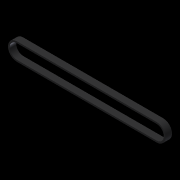
# Autodesk Inventor part: 150T 5mm GT2 Belt
Saved by Autodesk Inventor 2014 SP1 (Build 180222100, 222)
## iProperties
Created: 2013-11-29
Part Number: 150T 5mm GT2 Belt
Material: Rubber, Black
Document SubType Name: Modeling
Designer: Rauhul Varma
Mass: 40.3136 g
Surface Area: 284.75 cm^2
Volume: 43.3479 cm^3
Density: 0.93 g/cm^3
Appearance: Rubber - Black
Author: Rauhul Varma
Autodesk Inventor part; units mm, degrees
ref_plane "YZ Plane" through (0, 0, 0) normal (1, 0, 0) x (0, 1, 0)
ref_plane "XZ Plane" through (0, 0, 0) normal (0, 1, 0) x (-1, 0, 0)
ref_plane "XY Plane" through (0, 0, 0) normal (0, 0, 1) x (1, 0, 0)
sketch "Sketch1" plane through (0, 0, 0) normal (0, 0, 1) x (1, 0, 0)
  arc A0 (0, -16.545) -> (0, 16.545) centre (0, 0) ccw construction
  arc A1 (0, -20.365) -> (0, 20.365) centre (0, 0) ccw construction
  line L0 (0, 0) -> (320.2761, 0) construction
  arc A2 (320.2761, 20.365) -> (320.2761, -20.365) centre (320.2761, 0) ccw construction
  arc A3 (320.2761, 16.545) -> (320.2761, -16.545) centre (320.2761, 0) ccw construction
  line L1 (0, -16.545) -> (320.2761, -16.545)
  line L2 (320.2761, -20.365) -> (0, -20.365)
  line L3 (0, 20.365) -> (320.2761, 20.365)
  line L4 (320.2761, 16.545) -> (0, 16.545)
  arc A4 (320.2761, -16.545) -> (320.2761, 16.545) centre (320.2761, 0) ccw
  arc A5 (320.2761, -20.365) -> (320.2761, 20.365) centre (320.2761, 0) ccw
  arc A6 (0, 16.545) -> (0, -16.545) centre (0, 0) ccw
  arc A7 (0, 20.365) -> (0, -20.365) centre (0, 0) ccw
  dimension "d0" = 33.09
  dimension "d1" = 3.82
  dimension "d2" = 320.2761
  constraints: 16 point on circle, 10 end point, 8 centre point, 6 tangent, 4 coincident, 2 equal radius, 2 parallel, 1 horizontal
  measures "d0" diameter of A0
  measures "d1" radial gap between concentric circles of A1 A0
  measures "d2" distance of L0.start L0.end
extrude "Extrusion1" add sketch "Sketch1" along normal blind 15
body "Solid1"
